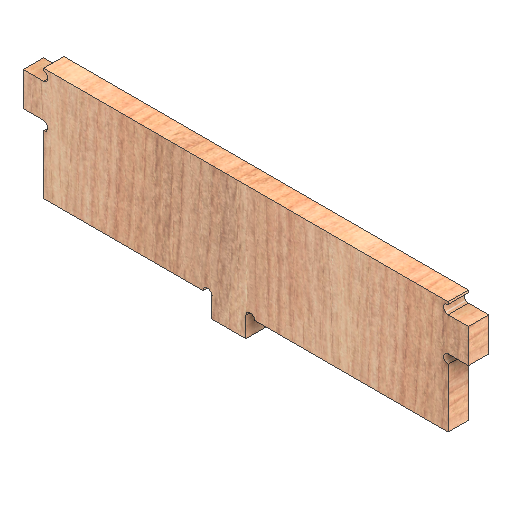
# Autodesk Inventor part: Layer 1 Plank
Saved by Autodesk Inventor 2021 (Build 250183000, 183)
## iProperties
Created: 2020-05-09
Part Number: Layer 1 Plank
Material: Wood (Birch)
Document SubType Name: Modeling
Designer: Dan Wikman
Density: 0.55 g/cm^3
Appearance: Birch - Natural Polished
Mass: 369.46 g
Surface Area: 935.816 cm^2
Volume: 671.746 cm^3
Autodesk Inventor part; units mm, degrees
ref_plane "YZ Plane" through (0, 0, 0) normal (1, 0, 0) x (0, 1, 0)
ref_plane "XZ Plane" through (0, 0, 0) normal (0, 1, 0) x (-1, 0, 0)
ref_plane "XY Plane" through (0, 0, 0) normal (0, 0, 1) x (1, 0, 0)
sketch "CONTOURS" plane through (0, 0, 0) normal (0, 0, 1) x (1, 0, 0)
  arc A0 (113.8436, 518.7397) -> (113.8436, 526.7397) centre (113.8436, 522.7397) ccw
  line L0 (113.8436, 526.7397) -> (113.8436, 528.7397)
  line L1 (113.8436, 528.7397) -> (472.3436, 528.7397)
  line L2 (472.3436, 528.7397) -> (472.3436, 526.7397)
  arc A1 (472.3436, 526.7397) -> (472.3436, 518.7397) centre (472.3436, 522.7397) ccw
  line L3 (472.3436, 518.7397) -> (490.3436, 518.7397)
  line L4 (490.3436, 518.7397) -> (490.3436, 488.7397)
  line L5 (490.3436, 488.7397) -> (472.3436, 488.7397)
  arc A2 (472.3436, 488.7397) -> (472.3436, 480.7397) centre (472.3436, 484.7397) ccw
  line L6 (472.3436, 480.7397) -> (472.3436, 428.7397)
  line L7 (472.3436, 428.7397) -> (301.0936, 428.7397)
  arc A3 (301.0936, 428.7397) -> (293.0936, 428.7397) centre (297.0936, 428.7397) ccw
  line L8 (293.0936, 428.7397) -> (293.0936, 410.7397)
  line L9 (293.0936, 410.7397) -> (263.0936, 410.7397)
  line L10 (263.0936, 410.7397) -> (263.0936, 428.7397)
  arc A4 (263.0936, 428.7397) -> (255.0936, 428.7397) centre (259.0936, 428.7397) ccw
  line L11 (255.0936, 428.7397) -> (113.8436, 428.7397)
  line L12 (113.8436, 428.7397) -> (113.8436, 480.7397)
  arc A5 (113.8436, 480.7397) -> (113.8436, 488.7397) centre (113.8436, 484.7397) ccw
  line L13 (113.8436, 488.7397) -> (95.8436, 488.7397)
  line L14 (95.8436, 488.7397) -> (95.8436, 518.7397)
  line L15 (95.8436, 518.7397) -> (113.8436, 518.7397)
  constraints: 32 end point, 12 point on circle, 6 centre point
extrude "Extrusion1" add sketch "CONTOURS" along normal blind 18
body "Solid1"
